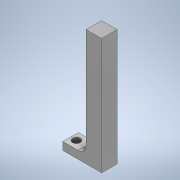
# Autodesk Inventor part: Bracket_Tall
Saved by Autodesk Inventor 2022 (Build 260153000, 153)
## iProperties
Created: 2022-11-11
Part Number: Bracket_Tall
Material: Aluminum, Anodized Silver
Document SubType Name: Modeling
Designer: bz72180
Density: 2.7 g/cm^3
Appearance: Anodized - Light Gray
Author: bz72180
Autodesk Inventor part; units mm, degrees
ref_plane "YZ Plane" through (0, 0, 0) normal (1, 0, 0) x (0, 1, 0)
ref_plane "XZ Plane" through (0, 0, 0) normal (0, 1, 0) x (-1, 0, 0)
ref_plane "XY Plane" through (0, 0, 0) normal (0, 0, 1) x (1, 0, 0)
sketch "Bracket Tall" plane through (0, 0, 0) normal (0, 0, 1) x (1, 0, 0)
  line L0 (0, 0) -> (30, 0)
  line L1 (25, 10) -> (0, 10)
  line L2 (0, 10) -> (0, 0)
  line L3 (30, 0) -> (55, 0)
  line L4 (55, 0) -> (55, 150)
  line L5 (55, 150) -> (35, 150)
  line L6 (35, 150) -> (35, 20)
  arc A0 (25, 10) -> (35, 20) centre (25, 20) ccw
  point P0 (35, 10)
  dimension "d0" = 35
  dimension "d2" = 20
  dimension "d3" = 150
  dimension "d4" = 10
  dimension "d10" = 10
  constraints: 14 end point, 3 parallel, 2 horizontal, 2 point on circle, 2 point on line, 2 tangent, 1 centre point, 1 perpendicular
  measures "d0" distance of point (35, 10) L1.end
  measures "d2" distance of L5.end L4.end
  measures "d3" distance of L4.end L3.end
  measures "d4" distance of L1.end L0.start
  measures "d10" radius of A0
extrude "Extrusion1" add sketch "Bracket Tall" along normal blind 20
sketch "Clearance Hole (M6-8)" plane through (0, 10, 0) normal (0, 1, 0) x (1, 0, 0)
  circle A0 centre (12.5, -10) radius 5
  line L0 (0, 0) -> (0, -20) projected
  line L1 (25, 0) -> (25, -20) projected
  dimension "d7" = 10
  constraints: 1 centre point
  measures "d7" diameter of A0
extrude "Extrusion2" cut sketch "Clearance Hole (M6-8)" against normal through all
sketch "Sketch3" plane through (0, 0, 0) normal (0, 0, -1) x (-1, 0, 0)
  line L0 (-55, 0) -> (-55, 150) projected
  line L1 (-55, 20) -> (-55, 0)
  circle A0 centre (-45, 20) radius 3
  line L2 (-45, 20) -> (-45, 130)
  point P0 (0, 0)
  dimension "d14" = 6
  dimension "d27" = 110
  constraints: 4 end point, 1 centre point, 1 vertical
  measures "d14" diameter of A0
  measures "d27" distance of L2.start L2.end
hole "Hole1" at (45, 20, 0) at (45, 130, 0) direction (0, 0, 1) diameter 3.242 depth 11.8 tip angle 118 thread size "M4x0.7" class "6H" standard "ANSI Metric M Profile"
move faces "Move1" translate (5, 0, 0) faces at (0, 6.6667, 6.6667)
body "Solid1"
